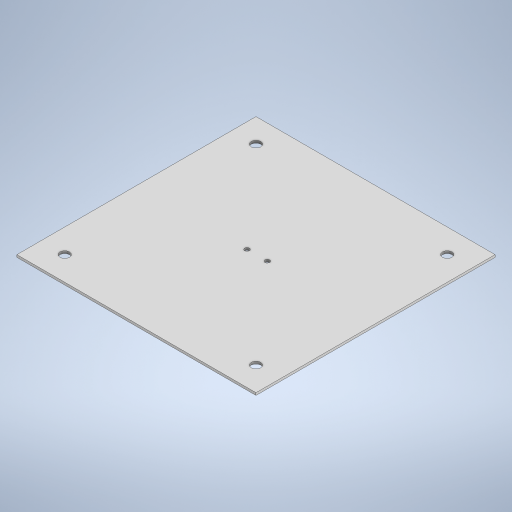
# Autodesk Inventor part: Пластина
Saved by Autodesk Inventor 2023 (Build 270158000, 158)
## iProperties
Created: 2022-05-06
Part Number: Пластина
Material: Типовые
Document SubType Name: Modeling
Designer: avkap
Density: 1 g/cm^3
Appearance: По умолчанию
Author: avkap
Autodesk Inventor part; units mm, degrees
ref_plane "YZ Plane" through (0, 0, 0) normal (1, 0, 0) x (0, 1, 0)
ref_plane "XZ Plane" through (0, 0, 0) normal (0, 1, 0) x (-1, 0, 0)
ref_plane "XY Plane" through (0, 0, 0) normal (0, 0, 1) x (1, 0, 0)
sketch "Эскиз1" plane through (0, 0, 0) normal (0, 1, 0) x (-1, 0, 0)
  line L0 (0, 0) -> (-200, 0)
  line L1 (-200, 0) -> (-200, -200)
  line L2 (-200, -200) -> (0, -200)
  line L3 (0, -200) -> (0, 0)
  line L4 (0, 0) -> (-20, 0)
  line L5 (-20, 0) -> (-20, -20)
  line L6 (-20, -20) -> (0, -20)
  line L7 (0, -20) -> (0, 0)
  line L8 (-200, -200) -> (-180, -200)
  line L9 (-180, -200) -> (-180, -180)
  line L10 (-180, -180) -> (-200, -180)
  line L11 (-200, -180) -> (-200, -200)
  line L12 (-180, -180) -> (-20, -180)
  line L13 (-20, -180) -> (-20, -20)
  line L14 (-20, -20) -> (-180, -20)
  line L15 (-180, -20) -> (-180, -180)
  circle A0 centre (-20, -20) radius 4
  circle A1 centre (-20, -180) radius 4
  circle A2 centre (-180, -20) radius 4
  circle A3 centre (-180, -180) radius 4
  line L16 (-200, -100) -> (0, -100)
  line L17 (-100, -100) -> (-92.5, -100)
  line L18 (-92.5, -100) -> (-109.5, -100)
  circle A4 centre (-92.5, -100) radius 2
  circle A5 centre (-109.5, -100) radius 2
  dimension "d0" = 200
  dimension "d1" = 200
  dimension "d2" = 20
  dimension "d3" = 20
  dimension "d4" = 20
  dimension "d5" = 20
  dimension "d6" = 8
  dimension "d7" = 8
  dimension "d8" = 8
  dimension "d9" = 8
  dimension "d10" = 7.5
  dimension "d11" = 17
  dimension "d12" = 4
  dimension "d13" = 4
  constraints: 38 end point, 8 parallel, 6 centre point, 6 coincident, 4 horizontal, 4 perpendicular, 3 midpoint, 2 point on line
  measures "d0" distance of L2.end L1.end
  measures "d1" distance of L1.end L0.end
  measures "d2" distance of L6.end L5.end
  measures "d3" distance of L5.end L4.end
  measures "d4" distance of L10.end L9.end
  measures "d5" distance of L9.end L8.end
  measures "d6" diameter of A0
  measures "d7" diameter of A1
  measures "d8" diameter of A2
  measures "d9" diameter of A3
  measures "d10" distance of L17.start L17.end
  measures "d11" distance of L17.end L18.end
  measures "d12" diameter of A4
  measures "d13" diameter of A5
extrude "Выдавливание1" add sketch "Эскиз1" along normal blind 2 contours L3 L6 A0 L5 L0 | L5 A0 L14 A2 L15 L16 L1 L0 | L3 L16 L13 A0 L6 | L3 L2 L9 A3 L12 A1 L13 L16 | L16 L15 A3 L10 L1 | A0 L13 L16 A4 A5 L15 A2 L14 | L13 A1 L12 A3 L15 L16 A5 A4 | L10 A3 L9 L2 L1
